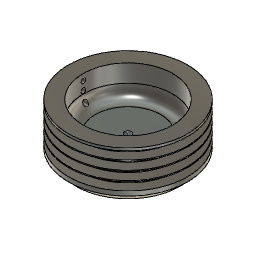
Test Rig v6 (Autodesk Fusion 360 archive; units mm, degrees)
design "Bearing Sleves (2)"
Autodesk Fusion 360 part; units mm, degrees
sketch "Sketch2" plane through (0, 0, 0) normal (0, 1, 0) x (1, 0, 0)
  line L0 (30, -10) -> (-30, -10)
  line L1 (-30, -10) -> (-30, 10)
  line L2 (-30, 10) -> (30, 10)
  line L3 (30, 10) -> (30, -10)
  line L4 (30, -10) -> (-30, 10) construction
  line L5 (-30, -10) -> (30, 10) construction
  line L6 (22.5, -10) -> (-22.5, -10)
  line L7 (-22.5, -10) -> (-22.5, 10)
  line L8 (-22.5, 10) -> (22.5, 10)
  line L9 (22.5, 10) -> (22.5, -10)
  line L10 (22.5, -10) -> (-22.5, 10) construction
  line L11 (-22.5, -10) -> (22.5, 10) construction
  line L12 (35, -8.75) -> (25, -8.75)
  line L13 (25, -8.75) -> (25, -4.75)
  line L14 (25, -4.75) -> (35, -4.75)
  line L15 (35, -4.75) -> (35, -8.75)
  line L16 (35, -8.75) -> (25, -4.75) construction
  line L17 (25, -8.75) -> (35, -4.75) construction
  line L18 (0, -10) -> (0, 10)
  line L19 (35, -0.25) -> (35, -4.25)
  line L20 (35, -4.25) -> (25, -4.25)
  line L21 (25, -4.25) -> (25, -0.25)
  line L22 (25, -0.25) -> (35, -0.25)
  line L23 (35, 4.25) -> (35, 0.25)
  line L24 (35, 0.25) -> (25, 0.25)
  line L25 (25, 0.25) -> (25, 4.25)
  line L26 (25, 4.25) -> (35, 4.25)
  line L27 (35, 8.75) -> (35, 4.75)
  line L28 (35, 4.75) -> (25, 4.75)
  line L29 (25, 4.75) -> (25, 8.75)
  line L30 (25, 8.75) -> (35, 8.75)
  line L31 (0, 0) -> (25, 0) construction
  line L32 (25, -0.25) -> (25, 0.25) construction
  line L33 (-2.5, -4.9) -> (2.5, -4.9)
  line L34 (2.5, -4.9) -> (2.5, 4.9)
  line L35 (2.5, 4.9) -> (-2.5, 4.9)
  line L36 (-2.5, 4.9) -> (-2.5, -4.9)
  line L37 (-2.5, -4.9) -> (2.5, 4.9) construction
  line L38 (2.5, -4.9) -> (-2.5, 4.9) construction
  line L39 (22.5, -4.9) -> (-22.5, -4.9)
  line L40 (22.5, 4.9) -> (-22.5, 4.9)
  point P0 (30, -6.75)
  point P1 (35, -2.25)
  point P2 (35, 2.25)
  point P3 (35, 6.75)
  dimension "d144_2" = 45
  dimension "d145_2" = 60
  dimension "d147_2" = 4
  dimension "d150_2" = 20
  dimension "d154_2" = -4.5
  dimension "d155_2" = 0
  dimension "d157_1" = 5
  dimension "d158_1" = 5.1
  dimension "d1" = 5
  constraint horizontal L0
  constraint perpendicular L0 L1
  constraint parallel L0 L2
  constraint parallel L1 L3
  constraint coincident L4 L31.start
  constraint coincident L5 L31.start
  constraint coincident L31.start origin
  constraint horizontal L6
  constraint perpendicular L6 L7
  constraint parallel L6 L8
  constraint parallel L7 L9
  constraint coincident L0 L6.start
  constraint coincident L10 L31.start
  constraint coincident L11 L31.start
  constraint horizontal L12
  constraint perpendicular L12 L13
  constraint parallel L12 L14
  constraint parallel L13 L15
  constraint coincident L16 P0
  constraint coincident L17 P0
  constraint coincident L3 P0
  constraint midpoint L0 L18.start
  constraint midpoint L8 L18.end
  constraint perpendicular L23 L31
  constraint midpoint L31.end L32
  constraint horizontal L33
  constraint perpendicular L33 L34
  constraint parallel L33 L35
  constraint parallel L34 L36
  constraint coincident L37 L31.start
  constraint coincident L38 L31.start
  constraint coincident L9 L39.start
  constraint coincident L7 L39.end
  constraint perpendicular L7 L39
  constraint coincident L9 L40.start
  constraint coincident L7 L40.end
  constraint perpendicular L7 L40
  constraint coincident L35.end L40
  constraint coincident L33.start L39
  constraint midpoint L19 P1
  constraint midpoint L23 P2
  constraint midpoint L27 P3
  measures "d144_2" distance of L7 L9
  measures "d145_2" distance of L0.start L0.end
  measures "d147_2" distance of L12.start L14.end
  measures "d150_2" distance of L0.end L1.end
  measures "d157_1" distance of L34 L36
  measures "d158_1" distance of L0 L39
  measures "d1" distance of L13 P0
revolve "Revolve1" add sketch "Sketch2" angle 360 about axis through (0, 0, 10) along (0, 0, -1) contours L0 L2 L3 L9 L12 L13 L14 L20 L21 L22 L24 L25 L26 L28 L29 L30 | L2 L8 L9 L18 L35 L40
sketch "Sketch3" plane through (0, 0, -4.9) normal (0, 0, 1) x (-1, 0, 0)
  circle A0 centre (0, 0) radius 22.5
hole "Hole1" at (0, 0, -4.9) direction (0, 0, -1) diameter 3.4 depth 6 tip angle 118
fillet "Fillet1" radius 6 1 edges at (-20.9774, -8.1363, -4.9)
move_face "OffsetFaces1" offset 2 1 faces at (20.4534, 1.5328, -10)
sketch "Sketch5" plane through (0, 0, -12) normal (0, 0, -1) x (1, 0, 0)
  circle A0 centre (0, 0) radius 1.7
  circle A1 centre (0, 0) radius 30
  circle A2 centre (0, 0) radius 6.35
  line L0 (0, 0) -> (-30, 0) construction
  line L1 (23.94, 3.81) -> (-23.94, 3.81)
  arc A3 (-23.94, 3.81) -> (-23.94, -3.81) centre (-23.94, 0) ccw
  line L2 (-23.94, -3.81) -> (23.94, -3.81)
  arc A4 (23.94, -3.81) -> (23.94, 3.81) centre (23.94, 0) ccw
  line L3 (23.94, 0) -> (-23.94, 0) construction
  line L4 (-24.3442, 3.7885) -> (-0.6737, 6.3142)
  line L5 (24.3442, 3.7885) -> (0.6737, 6.3142)
  line L6 (-27.75, 0) -> (27.75, 0) construction
  line L7 (-24.3442, -3.7885) -> (-0.6737, -6.3142)
  line L8 (0.6737, -6.3142) -> (24.3442, -3.7885)
  dimension "d8" = 12.7
  dimension "d9" = 55.5
  dimension "d10" = 7.62
  constraint concentric A0 A2
  constraint coincident A0.centre A1.centre
  constraint coincident A1 L0.end
  constraint horizontal L0
  constraint tangent L1 A3
  constraint tangent A3 L2
  constraint parallel L1 L2
  constraint tangent L2 A4
  constraint tangent L1 A4
  constraint coincident L0 A3.centre
  constraint parallel L0 L3
  constraint midpoint L3 A0.centre
  constraint coincident A3 L4.start
  constraint coincident A2 L4.end
  constraint tangent A2 L4
  constraint coincident A4 L5.start
  constraint coincident A2 L5.end
  constraint tangent A2 L5
  constraint tangent A4 L5
  constraint tangent A3 L4
  constraint midpoint A3 L6.start
  constraint midpoint A4 L6.end
  constraint coincident A3 L7.start
  constraint coincident A2 L7.end
  constraint coincident A2 L8.start
  constraint coincident A4 L8.end
  constraint tangent A4 L8
  constraint tangent A2 L8
  constraint tangent A2 L7
  constraint tangent A3 L7
  measures "d8" diameter of A2
  measures "d9" distance of L6.start L6.end
  measures "d10" distance of L1 L2
extrude "Extrude1" add sketch "Sketch5" along normal blind 3 contours A1
chamfer "Chamfer1" distance 4 angle 45 1 edges at (-27.9698, 10.8485, -15)
sketch "Sketch6" plane through (0, 0, 0) normal (1, 0, 0) x (0, 1, 0)
  line L0 (0, 15) -> (0, -15) construction
  line L1 (0, -8.75) -> (0, -4.75)
  line L2 (0, -4.25) -> (0, -0.25)
  line L3 (0, 0.8429) -> (0, 4.25)
  line L4 (0, 4.75) -> (0, 8.75)
  line L5 (30, 8.75) -> (-30, 8.75)
  line L6 (30, 4.75) -> (-30, 4.75)
  line L7 (30, 4.25) -> (-30, 4.25)
  line L8 (30, -4.25) -> (-30, -4.25)
  line L9 (30, -0.25) -> (-30, -0.25)
  line L10 (30, -4.75) -> (-30, -4.75)
  line L11 (30, -8.75) -> (-30, -8.75)
  line L12 (-3.3332, -15) -> (-26, -15)
  line L13 (26, -15) -> (3.3332, -15)
  point P0 (0, 6.75)
  point P1 (0, 2.5465)
  point P2 (0, -2.25)
  point P3 (0, -6.75)
  constraint vertical L0
  constraint midpoint origin L0
  constraint coincident L0 L1.start
  constraint coincident L0 L1.end
  constraint parallel L0 L1
  constraint coincident L0 L2.start
  constraint coincident L0 L2.end
  constraint coincident L0 L3.start
  constraint coincident L0 L3.end
  constraint coincident L0 L4.start
  constraint coincident L0 L4.end
  constraint coincident L4.end L5
  constraint coincident L4.start L6
  constraint coincident L3.end L7
  constraint coincident L2.start L8
  constraint coincident L2.end L9
  constraint coincident L1.end L10
  constraint coincident L1.start L11
  constraint midpoint L4 P0
  constraint midpoint L3 P1
  constraint midpoint L2 P2
  constraint midpoint L1 P3
hole "Hole2" at (0, 0, 6.75) at (0, 0, 2.5465) at (0, 0, -2.25) at (0, 0, -6.75) direction (-1, 0, 0) diameter 2.4 end through all
sketch "Sketch7" plane through (0, 0, -15) normal (0, 0, -1) x (1, 0, 0)
  arc A0 (-25.7855, -3.3332) -> (-24.3442, -3.7885) centre (-23.94, 0) ccw
  line L0 (-24.3442, 3.7885) -> (-0.6737, 6.3142)
  arc A1 (0.6737, 6.3142) -> (-0.6737, 6.3142) centre (0, 0) ccw
  line L1 (0.6737, 6.3142) -> (24.3442, 3.7885)
  arc A2 (24.3442, -3.7885) -> (25.7855, -3.3332) centre (23.94, 0) ccw
  line L2 (24.3442, -3.7885) -> (0.6737, -6.3142)
  arc A3 (-0.6737, -6.3142) -> (0.6737, -6.3142) centre (0, 0) ccw
  line L3 (-0.6737, -6.3142) -> (-24.3442, -3.7885)
  arc A4 (0.992, 9.2972) -> (-0.992, 9.2972) centre (0, 0) ccw
  line L4 (-24.6625, 6.7716) -> (-0.992, 9.2972)
  arc A5 (-24.6625, 6.7716) -> (-24.6625, -6.7716) centre (-23.94, 0) ccw
  line L5 (-0.992, -9.2972) -> (-24.6625, -6.7716)
  arc A6 (-0.992, -9.2972) -> (0.992, -9.2972) centre (0, 0) ccw
  line L6 (24.6625, -6.7716) -> (0.992, -9.2972)
  arc A7 (24.6625, -6.7716) -> (24.6625, 6.7716) centre (23.94, 0) ccw
  line L7 (0.992, 9.2972) -> (24.6625, 6.7716)
  circle A8 centre (0, 0) radius 23.5
  arc A9 (-25.7855, -3.3332) -> (25.7855, -3.3332) centre (0, 0) ccw
  arc A10 (25.7855, 3.3332) -> (-25.7855, 3.3332) centre (0, 0) ccw
  arc A11 (-24.3442, 3.7885) -> (-25.7855, 3.3332) centre (-23.94, 0) ccw
  arc A12 (25.7855, 3.3332) -> (24.3442, 3.7885) centre (23.94, 0) ccw
  constraint concentric A1 A4
  constraint parallel L0 L4
  constraint concentric A0 A5
  constraint parallel L3 L5
  constraint concentric A3 A6
  constraint parallel L2 L6
  constraint concentric A2 A7
  constraint parallel L1 L7
  constraint tangent L6 A7
  constraint tangent A6 L6
  constraint tangent L5 A6
  constraint tangent A5 L5
  constraint concentric A8 A9
extrude "Extrude2" cut sketch "Sketch7" against normal blind 4 contours L5 A6 L6 A8 | A4 L4 L7 A8
